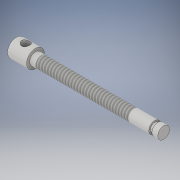
# Autodesk Inventor part: VS-004 (VISE SCREW)
Saved by Autodesk Inventor 2017 (Build 210142000, 142)
## iProperties
Created: 2016-11-30
Part Number: VS-004 (VISE SCREW)
Material: Generic
Document SubType Name: Modeling
Designer: SCC
Density: 1 g/cm^3
Appearance: Default
Author: SCC
Autodesk Inventor part; units mm, degrees
ref_plane "YZ Plane" through (0, 0, 0) normal (1, 0, 0) x (0, 1, 0)
ref_plane "XZ Plane" through (0, 0, 0) normal (0, 1, 0) x (-1, 0, 0)
ref_plane "XY Plane" through (0, 0, 0) normal (0, 0, 1) x (1, 0, 0)
sketch "Sketch1" plane through (0, 0, 0) normal (0, 0, 1) x (1, 0, 0)
  line L0 (0, 0) -> (0, 9.525)
  line L1 (0, 9.525) -> (20.6375, 9.525)
  line L2 (20.6375, 9.525) -> (20.6375, 6.35)
  line L3 (149.1107, 6.35) -> (149.1107, 4.7625)
  line L4 (149.1107, 4.7625) -> (152.4, 4.7625)
  line L5 (152.4, 4.7625) -> (152.4, 6.35)
  line L6 (152.4, 6.35) -> (158.75, 6.35)
  line L7 (158.75, 6.35) -> (158.75, 0)
  line L8 (158.75, 0) -> (0, 0)
  line L9 (149.1107, 6.35) -> (127, 6.35)
  line L10 (127, 6.35) -> (26.9875, 6.35)
  line L11 (26.9875, 6.35) -> (20.6375, 6.35)
  dimension "d0" = 9.525
  dimension "d1" = 20.6375
  dimension "d2" = 158.75
  dimension "d4" = 6.35
  dimension "d7" = 4.7625
  dimension "d8" = 3.2893
  dimension "d10" = 6.35
  dimension "d11" = 100.0125
  dimension "d12" = 6.35
  constraints: 24 end point, 7 perpendicular, 1 collinear, 1 horizontal, 1 point on line, 1 vertical
  measures "d0" distance of L0.start L0.end
  measures "d1" distance of L0.end L1.end
  measures "d2" distance of L7.end L0.start
  measures "d4" distance of L5.end L6.end
  measures "d7" distance between parallel lines of L8 L4
  measures "d8" distance between parallel lines of L3 L5
  measures "d10" distance of L10.end L2.end
  measures "d11" distance of L9.end L10.end
  measures "d12" distance between parallel lines of L8 L10
revolve "Revolution1" add sketch "Sketch1" angle 360 about axis through (158.75, 0, 0) along (-1, 0, 0)
thread "Thread1" size "5/8-8 Acme" class "2G" standard "Acme Threads" length 100.0125 offset 22.1107
sketch "Sketch2" plane through (0, 0, 0) normal (0, 1, 0) x (-1, 0, 0)
  circle A0 centre (-10.3188, 0) radius 4.3656
  line L0 (0, 9.525) -> (0, -9.525) projected
  point P0 (0, 0)
  dimension "d15" = 8.7312
  dimension "d27" = 10.3187
  dimension "d28" = 9.525
  constraints: 1 centre point
  measures "d15" diameter of A0
  measures "d27" distance from line of L0 A0.centre
  measures "d28" vertical distance of L0.start A0.centre
hole "Hole1" at (10.3188, 0, 0) direction (0, 1, 0) diameter 8.7313 end through all
sketch "Sketch3" plane through (0, 0, 0) normal (0, 1, 0) x (-1, 0, 0)
  circle A0 centre (-10.3188, 0) radius 4.3656
  line L0 (0, 9.525) -> (0, -9.525) projected
  point P0 (0, 0)
  dimension "d23" = 10.3187
  dimension "d24" = 8.7312
  dimension "d26" = 9.525
  constraints: 1 centre point
  measures "d23" distance from line of L0 A0.centre
  measures "d24" diameter of A0
  measures "d26" vertical distance of L0.start A0.centre
hole "Hole2" at (10.3188, 0, 0) direction (0, -1, 0) diameter 8.7313 end through all
body "Solid1"
